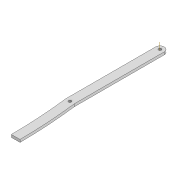
# Autodesk Inventor part: Part_3_p2
Saved by Autodesk Inventor 2022 (Build 260153000, 153)
## iProperties
Created: 2022-04-22
Part Number: Part_3_p2
Material: Generic
Document SubType Name: Modeling
Designer: dell
Density: 1 g/cm^3
Appearance: Default
Mass: 3.16709 g
Surface Area: 28.078 cm^2
Volume: 3.16709 cm^3
Author: dell
Autodesk Inventor part; units mm, degrees
ref_plane "YZ Plane" through (0, 0, 0) normal (1, 0, 0) x (0, 1, 0)
ref_plane "XZ Plane" through (0, 0, 0) normal (0, 1, 0) x (-1, 0, 0)
ref_plane "XY Plane" through (0, 0, 0) normal (0, 0, 1) x (1, 0, 0)
sketch "Sketch1" plane through (0, 0, 0) normal (0, 1, 0) x (-1, 0, 0)
  line L0 (0, 0) -> (0, -322.934) construction
  line L1 (5, 0) -> (5, -322.934)
  line L2 (-5, -322.934) -> (-5, 0)
  arc A0 (5, 0) -> (-5, 0) centre (0, 0) ccw
  arc A1 (-5, -322.934) -> (5, -322.934) centre (0, -322.934) ccw
  circle A2 centre (0, 0) radius 1.65
  circle A3 centre (0, -322.934) radius 1.65
  circle A4 centre (0, -74.182) radius 1.65
  circle A5 centre (0, -218.733) radius 1.65
  arc A6 (5, -74.182) -> (5, -218.733) centre (600.631, -146.4575) ccw
  arc A7 (-5, -74.182) -> (-5, -218.733) centre (590.631, -146.4575) ccw
  point P0 (0, -161.467)
  dimension "d0" = 3.3
  dimension "d1" = 3.3
  dimension "d2" = 10
  dimension "d3" = 322.934
  dimension "d4" = 3.3
  dimension "d5" = 74.182
  dimension "d8" = 3.3
  dimension "d9" = 218.733
  dimension "d12" = 600
  dimension "d13" = 600
  constraints: 8 centre point, 8 end point, 8 point on circle, 6 point on line, 4 horizontal alignment, 4 tangent, 2 coincident, 1 midpoint, 1 parallel, 1 vertical
  measures "d0" diameter of A2
  measures "d1" diameter of A3
  measures "d2" distance between parallel lines of L2 L1
  measures "d3" distance of L0.end L0.start
  measures "d4" diameter of A4
  measures "d5" distance of L0.start A4.centre
  measures "d8" diameter of A5
  measures "d9" distance of L0.start A5.centre
  measures "d12" radius of A6
  measures "d13" radius of A7
extrude "Extrusion1" add sketch "Sketch1" along normal blind 3 contours L1 A6 A1 L2 A0 | L2 A7
sketch "Sketch2" plane through (0, 3, 0) normal (0, 1, 0) x (1, 0, 0)
  line L0 (-80.742, 377.6004) -> (86.5972, 377.6004)
  line L1 (86.5972, 377.6004) -> (86.5972, -99.7148)
  line L2 (86.5972, -99.7148) -> (-80.742, -99.7148)
  line L3 (-80.742, -99.7148) -> (-80.742, 377.6004)
  line L4 (-25.6776, 342.7032) -> (34.5594, 342.7032)
  line L5 (34.5594, 342.7032) -> (34.5594, 151.6448)
  line L6 (34.5594, 151.6448) -> (-25.6776, 151.6448)
  line L7 (-25.6776, 151.6448) -> (-25.6776, 342.7032)
  point P0 (0, 0)
  constraints: 16 end point, 4 parallel, 2 horizontal, 2 perpendicular
extrude "Extrusion2" cut sketch "Sketch2" against normal blind 100
body "Solid1"
